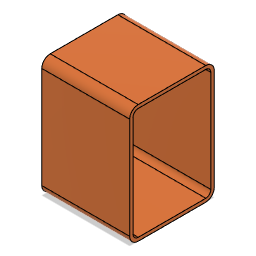
Контейнер v3 (Autodesk Fusion 360 design; units mm, degrees)
Autodesk Fusion 360 part; units mm, degrees
sketch "Sketch1" plane through (0, 0, 0) normal (1, 0, 0) x (0, 1, 0)
  line L0 (0, 0) -> (-70, 0)
  line L1 (-70, 0) -> (-70, 50)
  line L2 (-70, 50) -> (0, 50)
  line L3 (0, 50) -> (0, 0)
  dimension "d1" = 70
  dimension "d2" = 50
  constraint horizontal L0
  constraint vertical L1
  constraint horizontal L2
  constraint vertical L3
  constraint coincident L0.start L3.end
  measures "d1" distance of L0.start L0.end
  measures "d2" distance of L0.start L2.end
extrude "Extrude1" add sketch "Sketch1" along normal blind 50
fillet "Fillet1" radius 5 4 edges at (25, 0, 50) (25, 0, 0) (25, -70, 0) (25, -70, 50)
shell "Shell1" thickness 2 removed faces 1 at (50, -45, 16.6667)
extrude "Extrude3" add 1 faces at (0, -45, 16.6667) along direction (-1, 0, 0) blind 2
extrude "Extrude4" cut 1 faces at (2, -25, 17.3333) along direction (-1, 0, 0) blind 3
